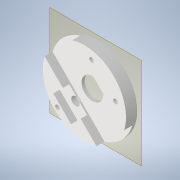
# Autodesk Inventor part: Matchboxscope_sample_v1
Saved by Autodesk Inventor 2022 (Build 260153000, 153)
## iProperties
Created: 2022-04-02
Part Number: Matchboxscope_sample_v1
Material: Generic
Document SubType Name: Modeling
Designer: Prakash Lab
Density: 1 g/cm^3
Appearance: Default
Author: Prakash Lab
Autodesk Inventor part; units mm, degrees
ref_plane "YZ Plane" through (0, 0, 0) normal (1, 0, 0) x (0, 1, 0)
ref_plane "XZ Plane" through (0, 0, 0) normal (0, 1, 0) x (-1, 0, 0)
ref_plane "XY Plane" through (0, 0, 0) normal (0, 0, 1) x (1, 0, 0)
ref_plane "Work Plane1" through (0, 0, 0) normal (0, 0, 1) x (1, 0, 0)
sketch "Sketch1" plane through (0, 0, 0) normal (0, 0, 1) x (1, 0, 0)
  circle A0 centre (0, 0) radius 25.9979
  circle A1 centre (-16.8291, -16.0481) radius 1.4
  circle A2 centre (19.4212, 5.2535) radius 1.4
  circle A3 centre (4.4725, 20.2023) radius 1.4
  circle A4 centre (-9.4998, -11.0022) radius 2.6601
  circle A5 centre (0.0001, -0.0022) radius 3.8801
  circle A6 centre (0.0001, -0.0022) radius 6.7754
  point P0 (0, 0)
extrude "Extrusion1" add sketch "Sketch1" along normal blind 7 contours A0
sketch "Sketch2" plane through (0, 0, 7) normal (0, 0, 1) x (1, 0, 0)
  line L0 (32.4435, -15.1193) -> (-15.1193, 32.4435)
  line L1 (-15.1193, 32.4435) -> (-32.4435, 15.1193)
  line L2 (-32.4435, 15.1193) -> (15.1193, -32.4435)
  line L3 (15.1193, -32.4435) -> (32.4435, -15.1193)
  line L4 (32.4435, -15.1193) -> (-32.4435, 15.1193) construction
  line L5 (-15.1193, 32.4435) -> (15.1193, -32.4435) construction
  line L6 (32.4435, -15.1193) -> (99.7074, -15.1193) construction
  point P0 (0, 0)
  dimension "d2" = 135
  dimension "d3" = 24.5
  constraints: 14 end point, 2 midpoint, 2 parallel, 1 equal length, 1 horizontal, 1 perpendicular
  measures "d2" angle of L6 L0
  measures "d3" distance of L1.end L0.end
extrude "Extrusion2" cut sketch "Sketch2" against normal blind 5
sketch "Sketch3" plane through (0, 0, 7) normal (0, 0, 1) x (1, 0, 0)
  line L0 (-8.3276, -20.7901) -> (-2.5509, -15.0135) projected
  line L1 (-2.5509, -15.0135) -> (-13.5111, -4.0533) projected
  line L2 (-19.2877, -9.8299) -> (-13.5111, -4.0533) projected
  line L3 (-8.3276, -20.7901) -> (-19.2877, -9.8299) projected
  line L4 (-13.5111, -3.9119) -> (-2.4095, -15.0135)
  line L5 (-2.4095, -15.0135) -> (-8.3276, -20.9315)
  line L6 (-8.3276, -20.9315) -> (-19.4292, -9.8299)
  line L7 (-19.4292, -9.8299) -> (-13.5111, -3.9119)
  line L8 (-8.9176, -8.4066) -> (-24.8767, 7.5526) projected
  line L9 (-13.4617, -3.8624) -> (-2.4095, -15.0135)
  line L10 (-2.4095, -15.0135) -> (-0.3384, -12.9607)
  line L11 (-0.3384, -12.9607) -> (-11.3905, -1.8096)
  line L12 (-11.3905, -1.8096) -> (-13.4617, -3.8624)
  line L13 (-13.4617, -3.8624) -> (-13.5111, -3.9119)
  line L14 (-8.9176, -8.4066) -> (-24.8767, 7.5526) projected
  point P0 (0, 0)
  dimension "d6" = 0.1
  constraints: 18 end point, 2 parallel, 2 perpendicular, 1 point on line, 3 other
  measures "d6" distance between parallel lines of L2 L7
extrude "Extrusion3" cut sketch "Sketch3" against normal blind 4 contours L3 L2 L1 L0 | L13 L9 L4 | L4 L5 L6 L7 | L9 L12 L11 L10
body "Solid1"
